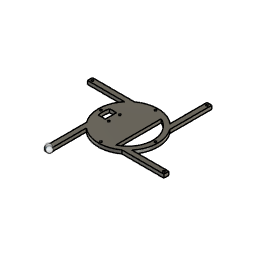
IR 支え v4 (Autodesk Fusion 360 design; units mm, degrees)
Autodesk Fusion 360 part; units mm, degrees
note: some values were not read from the file. Set by a fixed rule: which sketch regions a step uses.
sketch "スケッチ1" plane through (0, 0, 0) normal (0, 0, 1) x (1, 0, 0)
  circle A0 centre (0, 0) radius 37
  circle A1 centre (0, 0) radius 42
  line L0 (0, 65) -> (28.613, 65)
  line L1 (50, 0) -> (50, -28.613)
  line L2 (0, -50) -> (-28.613, -50)
  line L3 (-50, 0) -> (-50, 28.613)
  line L4 (-50, 28.613) -> (-30.7457, 28.613)
  line L5 (-30.7457, 28.613) -> (-85.2927, 28.613)
  line L6 (-28.613, -50) -> (-28.613, -30.7457)
  line L7 (-28.613, -30.7457) -> (-28.613, -85.2927)
  line L8 (50, -28.613) -> (30.7457, -28.613)
  line L9 (30.7457, -28.613) -> (85.2927, -28.613)
  line L10 (28.613, 65) -> (28.613, 30.7457)
  line L11 (28.613, 30.7457) -> (28.613, 85.2927)
  line L12 (-85.2927, 28.613) -> (-85.2927, 33.613)
  line L13 (-85.2927, 33.613) -> (-25.1827, 33.613)
  line L14 (28.613, 85.2927) -> (33.613, 85.2927)
  line L15 (33.613, 85.2927) -> (33.613, 25.1827)
  line L16 (85.2927, -28.613) -> (85.2927, -33.613)
  line L17 (85.2927, -33.613) -> (25.1827, -33.613)
  line L18 (-28.613, -85.2927) -> (-33.613, -85.2927)
  line L19 (-33.613, -85.2927) -> (-33.613, -25.1827)
  line L20 (-85.2927, 33.613) -> (-80.2927, 33.613)
  line L21 (-85.2927, 31.113) -> (-82.7927, 31.113)
  circle A2 centre (-82.7927, 31.113) radius 1.5
  line L22 (31.113, 85.2927) -> (31.113, 82.7927)
  circle A3 centre (31.113, 82.7927) radius 1.5
  line L23 (85.2927, -31.113) -> (82.7927, -31.113)
  line L24 (-31.113, -85.2927) -> (-31.113, -82.7927)
  circle A4 centre (-31.113, -82.7927) radius 1.5
  circle A5 centre (82.7927, -31.113) radius 1.5
  dimension "d1" = 74
  dimension "d2" = 84
  dimension "d3" = 28.613
  dimension "d4" = 28.613
  dimension "d5" = 28.613
  dimension "d6" = 28.613
  dimension "d7" = 54.547
  dimension "d8" = 54.547
  dimension "d9" = 54.547
  dimension "d10" = 54.547
  dimension "d11" = 5
  dimension "d12" = 5
  dimension "d13" = 5
  dimension "d14" = 5
  dimension "d15" = 5
  dimension "d16" = 3
  dimension "d17" = 2.5
  dimension "d18" = 3
  dimension "d19" = 2.5
  dimension "d20" = 2.5
  dimension "d21" = 3
  dimension "d22" = 3
  constraint coincident A0.centre A1.centre
  constraint horizontal L0
  constraint vertical L1
  constraint horizontal L2
  constraint vertical L3
  constraint coincident A1 L4.end
  constraint perpendicular L3 L4
  constraint perpendicular L3 L5
  constraint coincident A1 L6.end
  constraint perpendicular L2 L6
  constraint perpendicular L2 L7
  constraint coincident A1 L8.end
  constraint perpendicular L1 L8
  constraint perpendicular L1 L9
  constraint coincident A1 L10.end
  constraint perpendicular L0 L10
  constraint perpendicular L0 L11
  constraint perpendicular L5 L12
  constraint coincident A1 L13.end
  constraint perpendicular L12 L13
  constraint perpendicular L11 L14
  constraint coincident A1 L15.end
  constraint perpendicular L14 L15
  constraint perpendicular L9 L16
  constraint coincident A1 L17.end
  constraint perpendicular L16 L17
  constraint perpendicular L7 L18
  constraint coincident A1 L19.end
  constraint perpendicular L17 L19
  constraint perpendicular L12 L20
  constraint midpoint L12 L21.start
  constraint perpendicular L12 L21
  constraint coincident L21.end A2.centre
  constraint midpoint L14 L22.start
  constraint perpendicular L14 L22
  constraint coincident L22.end A3.centre
  constraint midpoint L16 L23.start
  constraint perpendicular L16 L23
  constraint midpoint L18 L24.start
  constraint perpendicular L18 L24
  constraint coincident L24.end A4.centre
  constraint coincident L23.end A5.centre
  measures "d1" diameter of A0
  measures "d2" diameter of A1
  measures "d3" distance of L0.start L0.end
  measures "d4" distance of L1.start L1.end
  measures "d5" distance of L2.start L2.end
  measures "d6" distance of L3.start L3.end
  measures "d7" distance of L4.end L5.end
  measures "d8" distance of L6.end L7.end
  measures "d9" distance of L8.end L9.end
  measures "d10" distance of L10.end L11.end
  measures "d11" distance of L5.end L12.end
  measures "d12" distance of L11.end L14.end
  measures "d13" distance of L9.end L16.end
  measures "d14" distance of L7.end L18.end
  measures "d15" distance of L12.end L20.end
  measures "d16" diameter of A2
  measures "d17" distance of L22.start L22.end
  measures "d18" diameter of A3
  measures "d19" distance of L23.start L23.end
  measures "d20" distance of L24.start L24.end
  measures "d21" diameter of A4
  measures "d22" diameter of A5
extrude "押し出し1" add sketch "スケッチ1" along normal blind 3
sketch "スケッチ2" plane through (0, 0, 0) normal (0, 0, 1) x (1, 0, 0)
  line L0 (0, 0) -> (0, 37)
  line L1 (0, 0) -> (37, 0)
  line L2 (0, 0) -> (-37, 0)
  line L3 (0, 0) -> (0, -37)
  line L4 (-37, 0) -> (-39.5, 0)
  line L5 (0, 37) -> (0, 39.5)
  line L6 (37, 0) -> (39.5, 0)
  line L7 (0, -37) -> (0, -39.5)
  circle A0 centre (0, -39.5) radius 1.5
  circle A1 centre (-39.5, 0) radius 1.5
  circle A2 centre (0, 39.5) radius 1.5
  circle A3 centre (39.5, 0) radius 1.5
  dimension "d25" = 37
  dimension "d26" = 37
  dimension "d27" = 37
  dimension "d28" = 37
  dimension "d30" = 2.5
  dimension "d31" = 2.5
  dimension "d32" = 2.5
  dimension "d33" = 2.5
  dimension "d34" = 3
  dimension "d35" = 3
  dimension "d36" = 3
  dimension "d37" = 3
  constraint coincident L0.start L1.start
  constraint vertical L0
  constraint perpendicular L0 L1
  constraint perpendicular L0 L2
  constraint perpendicular L2 L3
  constraint parallel L2 L4
  constraint parallel L0 L5
  constraint parallel L1 L6
  constraint parallel L3 L7
  constraint coincident L7.end A0.centre
  constraint coincident L4.end A1.centre
  constraint coincident L5.end A2.centre
  constraint coincident L6.end A3.centre
  measures "d25" distance of L0.start L0.end
  measures "d26" distance of L0.start L1.end
  measures "d27" distance of L0.start L2.end
  measures "d28" distance of L0.start L3.end
  measures "d30" distance of L2.end L4.end
  measures "d31" distance of L0.end L5.end
  measures "d32" distance of L1.end L6.end
  measures "d33" distance of L3.end L7.end
  measures "d34" diameter of A0
  measures "d35" diameter of A1
  measures "d36" diameter of A2
  measures "d37" diameter of A3
extrude "押し出し2" cut sketch "スケッチ2" along normal blind 3
sketch "スケッチ3" plane through (0, 0, 0) normal (0, 0, 1) x (1, 0, 0)
  line L0 (-31.1, -82.8) -> (-31.1, -83.7)
  line L1 (-31.1, -82.8) -> (-31.1, -86.8)
  line L2 (-31.1, -86.8) -> (-27.1, -86.8)
  constraint vertical L0
  constraint parallel L0 L1
  constraint perpendicular L1 L2
sketch "スケッチ4" plane through (0, 0, 0) normal (0, 0, 1) x (1, 0, 0)
  circle A0 centre (-82.8, 31.1) radius 1.5
  line L0 (-82.8, 27.6) -> (-86.3, 27.6)
  line L1 (-86.3, 27.6) -> (-86.3, 34.6)
  line L2 (-86.3, 34.6) -> (-82.8171, 34.6)
  line L3 (-39.5, 0) -> (-36, 0)
  line L4 (-39.5, 0) -> (-43, 0)
  circle A1 centre (0, 0) radius 36
  line L5 (31.1, 82.8) -> (34.6, 82.8)
  line L6 (34.6, 82.8) -> (34.6, 86.3)
  line L7 (34.6, 86.3) -> (27.6, 86.3)
  line L8 (82.8, -31.1) -> (86.3, -31.1)
  line L9 (86.3, -31.1) -> (86.3, -34.6)
  line L10 (86.3, -31.1) -> (86.3, -27.6)
  line L11 (-31.1, -82.8) -> (-31.1, -86.8)
  line L12 (-31.1, -82.8) -> (-31.1, -86.3)
  line L13 (-31.1, -86.3) -> (-27.6, -86.3)
  line L14 (-31.1, -86.3) -> (-34.6, -86.3)
  line L15 (-82.8, 27.6) -> (-32.9733, 27.6)
  line L16 (-82.8171, 34.6) -> (-25.5312, 34.6)
  line L17 (27.6, 86.3) -> (27.6, 85.5502)
  line L18 (27.6, 85.5502) -> (27.6, 32.9733)
  line L19 (34.6, 82.8) -> (34.6, 25.5312)
  line L20 (86.3, -27.6) -> (32.9733, -27.6)
  line L21 (86.3, -34.6) -> (25.5312, -34.6)
  line L22 (-27.6, -86.3) -> (-27.6, -32.9733)
  line L23 (-34.6, -86.3) -> (-34.6, -25.5312)
  arc A2 (-32.9733, 27.6) -> (-34.6, -25.5312) centre (0, 0) ccw
  arc A3 (27.6, 32.9733) -> (-25.5312, 34.6) centre (0, 0) ccw
  arc A4 (32.9733, -27.6) -> (34.6, 25.5312) centre (0, 0) ccw
  arc A5 (-27.6, -32.9733) -> (25.5312, -34.6) centre (0, 0) ccw
  circle A6 centre (0, 0) radius 42
  circle A7 centre (0, 0) radius 37
  line L24 (-82.8, 31.1) -> (-82.8, 28.6)
  line L25 (-82.8, 28.6) -> (-30.7578, 28.6)
  line L26 (-82.8, 31.1) -> (-82.8, 33.6)
  circle A8 centre (-31.1, -82.8) radius 1.5
  circle A9 centre (82.8, -31.1) radius 1.5
  circle A10 centre (31.1, 82.8) radius 1.5
  circle A11 centre (39.5, 0) radius 1.5
  circle A12 centre (0, 39.5) radius 1.5
  circle A13 centre (-39.5, 0) radius 1.5
  circle A14 centre (0, -39.5) radius 1.5
  dimension "d40" = 7
  dimension "d42" = 7
  dimension "d43" = 84
  dimension "d44" = 2.5
  dimension "d45" = 3
  constraint perpendicular L0 L1
  constraint horizontal L3
  constraint horizontal L4
  constraint coincident A1.centre A2.centre
  constraint coincident L3.end A1
  constraint perpendicular L5 L6
  constraint perpendicular L6 L7
  constraint horizontal L8
  constraint perpendicular L8 L9
  constraint perpendicular L8 L10
  constraint vertical L11
  constraint coincident L11 L12.end
  constraint perpendicular L12 L13
  constraint perpendicular L12 L14
  constraint parallel L2 L16
  constraint perpendicular L7 L17
  constraint parallel L17 L18
  constraint perpendicular L5 L19
  constraint perpendicular L10 L20
  constraint perpendicular L9 L21
  constraint perpendicular L13 L22
  constraint perpendicular L13 L23
  constraint concentric A2 A6
  constraint concentric A2 A7
  constraint coincident A0.centre L24.start
  constraint vertical L24
  constraint coincident A6 L25.end
  constraint perpendicular L24 L25
  constraint perpendicular L2 L26
  constraint coincident L11.start L12.start
  constraint coincident L8.start A9.centre
  constraint coincident L5.start A10.centre
  constraint coincident L3.start L4.start
  measures "d40" distance of L0.end L1.end
  measures "d42" distance of L6.end L7.end
  measures "d43" diameter of A6
  measures "d44" distance of A0.centre L26.end
  measures "d45" diameter of A9
extrude "押し出し3" add sketch "スケッチ4" against normal blind 5 contours L0 L1 L2 L6 L7 L9 L10 L13 L14 L15 L16 L17 L18 L19 L20 L21 L22 L23 A2 A3 A4 A5 | A6 | A7
extrude "押し出し4" cut 1 faces at (-45.9464, 31.5175, 3) along direction (0, 0, -1) blind 3
sketch "スケッチ5" plane through (0, 0, 0) normal (0, 0, 1) x (1, 0, 0)
  line L0 (15, 33) -> (15, -33)
  arc A0 (15, 32.7261) -> (15, -32.7261) centre (0, 0) ccw
  dimension "d50" = 36
  constraint vertical L0
  constraint coincident L0 A0.start
  constraint coincident L0 A0.end
  constraint coincident A0.centre origin
  measures "d50" radius of A0
extrude "押し出し5" add sketch "スケッチ5" against normal blind 5
sketch "スケッチ6" plane through (0, 0, 0) normal (0, 0, 1) x (1, 0, 0)
  line L0 (0, 0) -> (-20, 0)
  circle A0 centre (-20, -8) radius 1.5
  circle A1 centre (-20, 8) radius 1.5
  circle A2 centre (0, 0) radius 36
  line L1 (-20, -8) -> (-35.0999, -8)
  line L2 (-20, 8) -> (-35.0999, 8)
  line L3 (-20, -8) -> (-25, -8)
  line L4 (-25, 8) -> (-25, -8)
  dimension "d53" = 8
  dimension "d54" = 8
  dimension "d55" = 3
  dimension "d56" = 3
  constraint coincident L0.start A2.centre
  constraint horizontal L0
  constraint coincident A1.centre L2.start
  constraint coincident A0.centre L1.start
  constraint coincident A2 L1.end
  constraint coincident A2 L2.end
  constraint coincident L1 L3.end
  constraint parallel L1 L3
  constraint coincident L2 L4.start
  constraint perpendicular L1 L4
  measures "d53" distance of L0.end A0.centre
  measures "d54" distance of L0.end A1.centre
  measures "d55" diameter of A0
  measures "d56" diameter of A1
extrude "押し出し6" cut sketch "スケッチ6" against normal blind 5 contours A0 | A1 | A2 L1 L2 L4 picked at (-28.6332, 0.8955)
